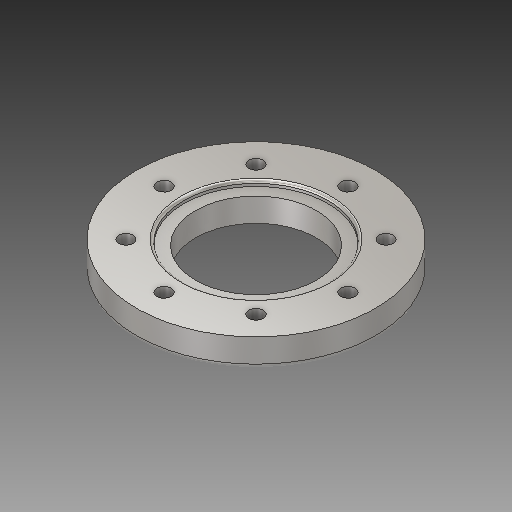
# Autodesk Inventor part: 301-06
Saved by Autodesk Inventor 2019 (Build 230136000, 136)
## iProperties
Company: Autodesk Inc.
Created: 2017-03-14
Part Number: 301-06
Material: Stainless Steel
Document SubType Name: Modeling
Designer: Autodesk Inc.
Density: 8 g/cm^3
Appearance: Semi-Polished
Mass: 378.172 g
Surface Area: 158.599 cm^2
Volume: 47.2716 cm^3
Author: Inventor
Autodesk Inventor part; units mm, degrees
ref_plane "YZ Plane" through (0, 0, 0) normal (1, 0, 0) x (0, 1, 0)
ref_plane "XZ Plane" through (0, 0, 0) normal (0, 1, 0) x (-1, 0, 0)
ref_plane "XY Plane" through (0, 0, 0) normal (0, 0, 1) x (1, 0, 0)
sketch "Sketch1" plane through (0, 0, 0) normal (0, 1, 0) x (-1, 0, 0)
  circle A0 centre (0, 0) radius 45.5
  dimension "d0" = 91
  constraints: 1 centre point, 1 coincident
  measures "d0" diameter of A0
extrude "Extrusion1" add sketch "Sketch1" along normal mid plane 11
fillet "Fillet1" radius 2 1 edges at (45.5, -5.5, 0)
hole "Hole1" at (0, 5.5, 0) direction (0, -1, 0) diameter 46 end through all
hole "Hole2" at (0, 5.5, 0) direction (0, -1, 0) diameter 55 depth 2
fillet "Fillet2" radius 1 1 edges at (0, 5.5, -27.5)
sketch "Sketch2" plane through (0, -5.5, 0) normal (0, 1, 0) x (1, 0, 0)
  line L0 (-35, 0) -> (0, 0) construction
  dimension "d23" = 35
  constraints: 2 end point, 1 horizontal
  measures "d23" distance of L0.start L0.end
hole "Hole3" at (-35, -5.5, 0) direction (0, 1, 0) diameter 5.5 end through all counterbore diameter 10 counterbore depth 5
pattern_circular "Circular Pattern2" count 8 over 360 about axis through (0, -123.6627, 0) along (0, 1, 0) of "Hole3"
body "Solid1"
